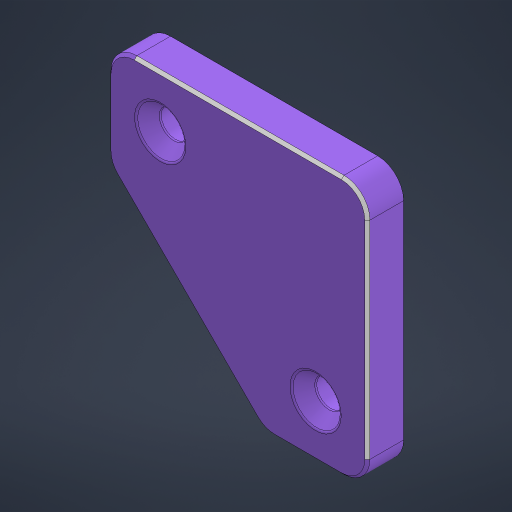
# Autodesk Inventor part: 모서리 결합 수정
Saved by Autodesk Inventor 2024 (Build 280153000, 153)
## iProperties
Created: 2024-01-11
Part Number: 모서리 결합 수정
Material: 일반
Document SubType Name: Modeling
Designer: KBU
Density: 1 g/cm^3
Appearance: 기본값
Author: KBU
Autodesk Inventor part; units mm, degrees
ref_plane "YZ Plane" through (0, 0, 0) normal (1, 0, 0) x (0, 1, 0)
ref_plane "XZ Plane" through (0, 0, 0) normal (0, 1, 0) x (-1, 0, 0)
ref_plane "XY Plane" through (0, 0, 0) normal (0, 0, 1) x (1, 0, 0)
sketch "스케치1" plane through (0, 0, 0) normal (0, 0, 1) x (1, 0, 0)
  line L0 (5, -25) -> (25, -25)
  line L1 (25, -25) -> (25, 25)
  line L2 (25, 25) -> (-25, 25)
  line L3 (-25, 25) -> (-25, 5)
  line L4 (-10, -10) -> (25, 25) construction
  line L5 (25, -25) -> (-25, 25) construction
  line L6 (5, -25) -> (-25, 5)
  point P0 (0, 0)
  dimension "d0" = 50
  dimension "d1" = 50
  dimension "d2" = 20
  dimension "d3" = 20
  constraints: 14 end point, 2 midpoint, 2 parallel, 1 horizontal, 1 perpendicular, 1 point on line
  measures "d0" distance of L0.end L1.end
  measures "d1" distance of L1.end L2.end
  measures "d2" distance from line of L3.end L2
  measures "d3" distance from line of L0.start L1
extrude "돌출1" add sketch "스케치1" along normal blind 7
sketch "스케치2" plane through (0, 0, 0) normal (0, 0, -1) x (-1, 0, 0)
  line L0 (25, 25) -> (25, 5) projected
  line L1 (-25, 25) -> (25, 25) projected
  line L2 (-25, -25) -> (-25, 25) projected
  line L3 (-5, -25) -> (-25, -25) projected
  line L4 (-15, 15) -> (15, 15) construction
  line L5 (-15, -15) -> (-15, 15) construction
  circle A0 centre (-15, -15) radius 2.7
  circle A1 centre (15, 15) radius 2.7
  point P0 (-7.0711, -25)
  point P1 (25, 7.0711)
  point P2 (25, 20)
  point P3 (20, 25)
  point P4 (-20, 25)
  point P5 (-25, 20)
  point P6 (-25, -20)
  point P7 (-20, -25)
  point P8 (0, 0)
  point P9 (-25, 0)
  dimension "d8" = 10
  dimension "d10" = 10
  dimension "d11" = 10
  dimension "d12" = 10
  dimension "d13" = 5.4
  dimension "d14" = 5.4
  constraints: 4 end point, 2 centre point, 2 coincident, 1 horizontal, 1 midpoint
  measures "d8" distance between parallel lines of L1 L4
  measures "d10" distance between parallel lines of L2 L5
  measures "d11" distance from line of L0 L4.end
  measures "d12" distance from line of L3 L5.start
  measures "d13" diameter of A0
  measures "d14" diameter of A1
extrude "돌출2" cut sketch "스케치2" against normal blind 10
chamfer "모따기2" distance 2 distance2 2.75 1 edges at (-12.3, 15, 7) measured on face at (-11.8, 15, 7)
fillet "모깎기3" radius 0.5 2 edges at (-12.3, 15, 4.25) (-10.3, 15, 7)
chamfer "모따기3" distance 2 distance2 2.75 1 edges at (17.7, -15, 7) measured on face at (18.2, -15, 7)
fillet "모깎기4" radius 0.5 2 edges at (19.7, -15, 7) (17.7, -15, 4.25)
sketch "스케치3" plane through (0, 0, 7) normal (0, 0, 1) x (1, 0, 0)
  line L0 (25, -25) -> (25, 25) projected
  line L1 (25, 25) -> (-25, 25) projected
  line L2 (-25, 25) -> (-25, 5) projected
  line L3 (5, -25) -> (25, -25) projected
  line L4 (-21, 21) -> (21, 21)
  line L5 (21, 21) -> (21, -21)
  line L6 (-21, 21) -> (-25, 21)
  line L7 (21, -21) -> (21, -25)
  point P0 (0, 0)
  dimension "d28" = 4
  constraints: 8 end point, 2 perpendicular, 2 point on line, 1 other
  measures "d28" distance between parallel lines of L1 L4
extrude "돌출3" [suppressed]
sketch "스케치4" plane through (0, 0, 12.3) normal (0, 0, 1) x (1, 0, 0)
  line L0 (-25, 25) -> (-25, 21) projected
  line L1 (21, -25) -> (25, -25) projected
  line L2 (25, -25) -> (25, 25) projected
  line L3 (25, 25) -> (-25, 25) projected
  line L4 (25, 25) -> (-25, 25)
  line L5 (-25, 21) -> (-25, 5) projected
  line L6 (-25, 5) -> (5, -25) projected
  line L7 (-25, 5) -> (5, -25)
  line L8 (5, -25) -> (25, -25)
  circle A0 centre (-15, 15) radius 5.2
  circle A1 centre (15, -15) radius 5.2 projected
  circle A2 centre (15, -15) radius 5.2
  point P0 (0, 0)
  point P1 (21, -25)
  constraints: 6 end point, 2 centre point, 2 collinear, 1 coincident, 1 parallel
extrude "돌출4" [suppressed]
chamfer "모따기4" [suppressed]
fillet "모깎기5" radius 5 5 edges at (25, 25, 3.5) (25, -25, 3.5) (-25, 25, 3.5) (5, -25, 3.5) (-25, 5, 3.5)
fillet "모깎기6" [suppressed]
chamfer "모따기5" distance 0.5 angle 45 7 edges at (13.5355, -25, 7) (23.5355, -23.5355, 7) (5.1577, -24.6194, 7) (-10, -10, 7) (-24.6194, 5.1577, 7) (-25, 13.5355, 7) (-23.5355, 23.5355, 7)
sketch "스케치6" plane through (0, 0, 0) normal (0, 0, -1) x (-1, 0, 0)
  arc A0 (23.5355, 3.5355) -> (25, 7.0711) centre (20, 7.0711) ccw projected
  line L0 (25, 20) -> (25, 7.0711) projected
  line L1 (-20, 25) -> (20, 25) projected
  line L2 (-25, -20) -> (-25, 20) projected
  line L3 (-7.0711, -25) -> (-20, -25) projected
  arc A1 (-7.0711, -25) -> (-3.5355, -23.5355) centre (-7.0711, -20) ccw projected
  line L4 (23.5355, 3.5355) -> (-3.5355, -23.5355) projected
  line L5 (-11.5, 11.5) -> (32.9305, 11.5)
  line L6 (32.9305, 11.5) -> (32.9305, -27.6838)
  line L7 (32.9305, -27.6838) -> (-11.5, -27.6838)
  line L8 (-11.5, -27.6838) -> (-11.5, 11.5)
  point P0 (0, 0)
  point P1 (25, 11.5)
  point P2 (-11.5, -25)
  dimension "d43" = 13.5
  dimension "d44" = 13.5
  constraints: 8 end point, 2 parallel, 1 horizontal, 1 perpendicular
  measures "d43" distance between parallel lines of L1 L5
  measures "d44" distance between parallel lines of L2 L8
extrude "돌출5" cut sketch "스케치6" against normal blind 5.3 contours L4 A1 L3 L8 L5 L0 A0
equation "\"d13\" = d14"
